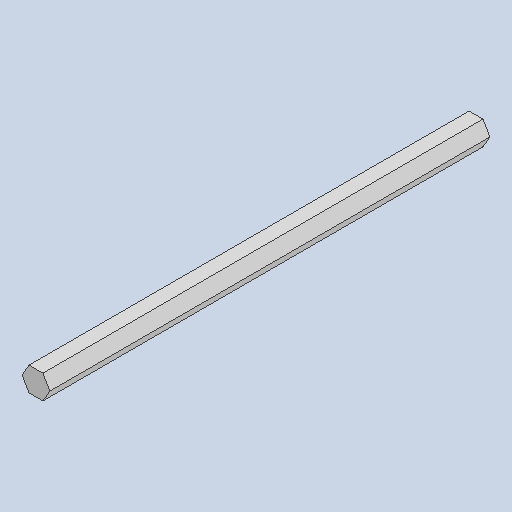
# Autodesk Inventor part: Eje_Entrada
Saved by Autodesk Inventor 2022 (Build 260153000, 153)
## iProperties
Created: 2022-02-21
Part Number: Eje_Entrada
Material: Generic
Document SubType Name: Modeling
Designer: katha
Density: 1 g/cm^3
Appearance: Default
Author: katha
Autodesk Inventor part; units mm, degrees
ref_plane "YZ Plane" through (0, 0, 0) normal (1, 0, 0) x (0, 1, 0)
ref_plane "XZ Plane" through (0, 0, 0) normal (0, 1, 0) x (-1, 0, 0)
ref_plane "XY Plane" through (0, 0, 0) normal (0, 0, 1) x (1, 0, 0)
sketch "Sketch1" plane through (0, 0, 0) normal (0, 0, 1) x (1, 0, 0)
  line L0 (-34.1536, 0) -> (-35.8268, 2.8981) projected
  line L1 (-35.8268, 2.8981) -> (-39.1732, 2.8981) projected
  line L2 (-39.1732, 2.8981) -> (-40.8464, 0) projected
  line L3 (-40.8464, 0) -> (-39.1732, -2.8981) projected
  line L4 (-39.1732, -2.8981) -> (-35.8268, -2.8981) projected
  line L5 (-35.8268, -2.8981) -> (-34.1536, 0) projected
  line L6 (-36, 2.5981) -> (-34.5, 0)
  line L7 (-34.5, 0) -> (-36, -2.5981)
  line L8 (-36, -2.5981) -> (-39, -2.5981)
  line L9 (-39, -2.5981) -> (-40.5, 0)
  line L10 (-40.5, 0) -> (-39, 2.5981)
  line L11 (-39, 2.5981) -> (-36, 2.5981)
  point P0 (0, 0)
  dimension "d0" = 0.3
  constraints: 12 end point, 5 other
  measures "d0" distance between parallel lines of L0 L6
extrude "Extrusion1" add sketch "Sketch1" along normal blind 95 contours L6 L7 L8 L9 L10 L11
body "Solid1"
